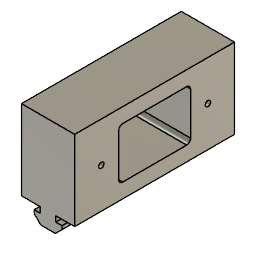
Govde (Autodesk Fusion 360 archive; units mm, degrees)
design "power_soket"
Autodesk Fusion 360 part; units mm, degrees
note: some values were not read from the file. Chosen so that the rebuilt part matches the saved one: which pieces of a blend or face edit are solid.
sketch "Sketch1" plane through (0, 0, 0) normal (0, 1, 0) x (1, 0, 0)
  line L0 (2.8825, -8.6547) -> (4.3945, -10.1667)
  line L1 (3.9, -0.21) -> (3.9, -2.8393)
  line L2 (-8.2, 5.5) -> (-8.2, 3.125)
  line L3 (-2.925, -8.676) -> (-4.4001, -10.1511)
  arc A0 (9.4998, -10.0253) -> (10.0042, -9.4999) centre (9.4925, -9.5135) ccw
  line L4 (0, -4.0611) -> (-0.1019, -4.163)
  line L5 (5.5, 8.2) -> (3.125, 8.2)
  line L6 (-6.5607, -5.5) -> (-8.2, -5.5)
  line L7 (5.2425, -6.658) -> (5.2425, -7.96)
  line L8 (-8.2, -5.5) -> (-8.2, -3.1249)
  line L9 (0, -4.0611) -> (0.1019, -4.163)
  line L10 (-2.7368, -4.163) -> (-5.2537, -6.6799)
  line L11 (-3.125, 8.545) -> (-4.58, 10)
  line L12 (6.5607, 5.5) -> (8.2, 5.5)
  line L13 (-3.125, 8.2) -> (-3.125, 8.545)
  arc A1 (-9.5, 10) -> (-10, 9.5) centre (-9.5, 9.5) ccw
  line L14 (8.2, 3.125) -> (8.545, 3.125)
  line L15 (-3.9, 0.21) -> (-3.9, 2.8393)
  line L16 (-10, 9.5) -> (-10, 4.58)
  line L17 (0.1019, -4.163) -> (2.7475, -4.163)
  line L18 (-3.125, -8.14) -> (-3.125, -8.5931)
  line L19 (-6.5607, 5.5) -> (-8.2, 5.5)
  line L20 (-5.2537, -7.94) -> (-2.925, -7.94)
  line L21 (3.69, 0) -> (3.9, -0.21)
  line L22 (-10.0013, -4.5807) -> (-10.0013, -9.5)
  line L23 (-0.1019, -4.163) -> (-2.7368, -4.163)
  line L24 (-3.69, 0) -> (-3.9, -0.21)
  line L25 (3.9, -2.8393) -> (6.5607, -5.5)
  line L26 (-5.4537, -6.5971) -> (-5.4537, -8.14)
  arc A2 (10, 9.5) -> (9.5, 10) centre (9.5, 9.5) ccw
  line L27 (-3.9, 2.8393) -> (-6.5607, 5.5)
  line L28 (8.545, 3.125) -> (10, 4.58)
  line L29 (10.0042, -4.5823) -> (10.0042, -9.4999)
  line L30 (-5.4537, -8.14) -> (-3.125, -8.14)
  line L31 (-10, -10.0258) -> (-10, -15)
  line L32 (-3.125, -8.5931) -> (-4.5415, -10.0097)
  line L33 (-3.9, -2.8393) -> (-6.5607, -5.5)
  line L34 (3.0825, -8.5719) -> (4.5359, -10.0253)
  line L35 (5.4425, -8.16) -> (3.0825, -8.16)
  line L36 (-2.925, -7.94) -> (-2.925, -8.676)
  line L37 (3.125, 8.2) -> (3.125, 8.545)
  line L38 (8.2, -3.1245) -> (8.5464, -3.1245)
  line L39 (8.2, -5.5) -> (8.2, -3.1245)
  line L40 (0, -3.7782) -> (0.1847, -3.963)
  line L41 (0, -3.7782) -> (-0.1847, -3.963)
  line L42 (0.1847, -3.963) -> (2.8304, -3.963)
  line L43 (-9.5, -10.0097) -> (-4.5415, -10.0097)
  line L44 (4.5359, -10.0253) -> (9.4998, -10.0253)
  line L45 (6.5607, -5.5) -> (8.2, -5.5)
  line L46 (-2.8196, -3.963) -> (-5.4537, -6.5971)
  line L47 (-8.2, -3.1249) -> (-8.5454, -3.1249)
  line L48 (8.5464, -3.1245) -> (10.0042, -4.5823)
  arc A3 (-10.0013, -9.5) -> (-9.5, -10.0097) centre (-9.4969, -9.5053) ccw
  line L49 (10, -15) -> (10, -10.0258)
  line L50 (-5.2537, -6.6799) -> (-5.2537, -7.94)
  line L51 (5.2425, -7.96) -> (2.8825, -7.96)
  line L52 (3.0825, -8.16) -> (3.0825, -8.5719)
  line L53 (5.4425, -6.5751) -> (5.4425, -8.16)
  line L54 (3.9, 0.21) -> (3.9, 2.8393)
  line L55 (-3.9, -0.21) -> (-3.9, -2.8393)
  line L56 (3.9, 2.8393) -> (6.5607, 5.5)
  line L57 (-5.5, 6.5607) -> (-5.5, 8.2)
  line L58 (2.8825, -7.96) -> (2.8825, -8.6547)
  line L59 (-8.5454, -3.1249) -> (-10.0013, -4.5807)
  line L60 (0, 3.69) -> (-0.21, 3.9)
  line L61 (2.8304, -3.963) -> (5.4425, -6.5751)
  line L62 (2.7475, -4.163) -> (5.2425, -6.658)
  line L63 (-8.545, 3.125) -> (-10, 4.58)
  line L64 (-0.1847, -3.963) -> (-2.8196, -3.963)
  line L65 (5.5, 6.5607) -> (5.5, 8.2)
  line L66 (-0.21, 3.9) -> (-2.8393, 3.9)
  line L67 (3.69, 0) -> (3.9, 0.21)
  line L68 (-5.5, 8.2) -> (-3.125, 8.2)
  line L69 (-8.2, 3.125) -> (-8.545, 3.125)
  line L70 (-2.8393, 3.9) -> (-5.5, 6.5607)
  line L71 (2.8393, 3.9) -> (5.5, 6.5607)
  line L72 (10, 9.5) -> (10, 4.58)
  line L73 (8.2, 5.5) -> (8.2, 3.125)
  line L74 (-3.69, 0) -> (-3.9, 0.21)
  line L75 (0.21, 3.9) -> (2.8393, 3.9)
  line L76 (4.58, 10) -> (9.5, 10)
  circle A4 centre (0, 0) radius 2.5
  line L77 (3.125, 8.545) -> (4.58, 10)
  line L78 (-9.5, 10) -> (-4.58, 10)
  line L79 (0, 3.69) -> (0.21, 3.9)
  line L80 (-10, -15) -> (10, -15)
  line L81 (0.1019, -4.163) -> (-0.1019, -4.163)
  line L82 (4.2531, -10.0253) -> (4.5359, -10.0253)
  line L83 (10, -10.0258) -> (4.2536, -10.0258)
  line L84 (-4.2748, -10.0258) -> (-10, -10.0258)
  line L85 (2.8825, -8.6547) -> (2.8825, -10.0258)
  line L86 (2.8825, -10.0258) -> (4.2536, -10.0258)
  line L87 (-2.925, -8.676) -> (-2.925, -10.0353)
  line L88 (-2.925, -10.0353) -> (-4.2748, -10.0258)
  point P0 (0, -10)
  dimension "d1" = 0.2
  dimension "d2" = 5
  constraint parallel L23 L81
  constraint coincident L0 L82.start
  constraint coincident L0 L83.end
  constraint coincident L3 L84.start
  constraint collinear L83 L84
  constraint perpendicular L35 L85
  constraint perpendicular L86 L87
  measures "d2" diameter of A4
extrude "Extrude1" add sketch "Sketch1" along normal blind 60 contours L7 L10 L17 L20 L23 L31 L36 L44 L49 L50 L51 L58 L62 L80 L81 L82 L83 L84 L85 L86 L87 L88
sketch "Sketch2" plane through (10, 0, 0) normal (1, 0, 0) x (0, 1, 0)
  line L0 (0, 15) -> (0, 10.0258)
  line L1 (0, 10.0258) -> (60, 10.0258)
  line L2 (60, 10.0258) -> (60, 15)
  line L3 (60, 15) -> (0, 15)
  line L4 (0, 10.0258) -> (60, 10.0258)
  line L5 (60, 10.0258) -> (60, 40.0258)
  line L6 (60, 40.0258) -> (0, 40.0258)
  line L7 (0, 40.0258) -> (0, 10.0258)
  line L8 (60, 40.0258) -> (0, 10.0258) construction
  line L9 (0, 40.0258) -> (60, 10.0258) construction
  line L10 (43.5, 34.5258) -> (16.5, 34.5258)
  line L11 (16.5, 34.5258) -> (16.5, 15.5258)
  line L12 (16.5, 15.5258) -> (43.5, 15.5258)
  line L13 (43.5, 15.5258) -> (43.5, 34.5258)
  line L14 (43.5, 34.5258) -> (16.5, 15.5258) construction
  line L15 (16.5, 34.5258) -> (43.5, 15.5258) construction
  line L16 (16.5, 25.0258) -> (10, 25.0258)
  line L17 (43.5, 25.0258) -> (50, 25.0258)
  circle A0 centre (10, 25.0258) radius 1
  circle A1 centre (50, 25.0258) radius 1
  point P0 (30, 25.0258)
  dimension "d5" = 30
  dimension "d6" = 60
  dimension "d7" = 27
  dimension "d8" = 19
  dimension "d9" = 6.5
  dimension "d10" = 6.5
  dimension "d11" = 2
  dimension "d12" = 2
  constraint horizontal L4
  constraint vertical L5
  constraint horizontal L6
  constraint vertical L7
  constraint coincident L0.end L1.start
  constraint horizontal L10
  constraint perpendicular L10 L11
  constraint parallel L10 L12
  constraint parallel L11 L13
  constraint coincident L14 P0
  constraint coincident L15 P0
  constraint midpoint L9 P0
  constraint midpoint L11 L16.start
  constraint perpendicular L11 L16
  constraint midpoint L13 L17.start
  constraint perpendicular L13 L17
  constraint coincident L16.end A0.centre
  constraint coincident L17.end A1.centre
  measures "d5" distance of L0.end L6.end
  measures "d6" distance of L5.end L6.end
  measures "d7" distance of L11.end L12.end
  measures "d8" distance of L10.end L11.end
  measures "d9" distance of L16.start L16.end
  measures "d10" distance of L17.start L17.end
  measures "d11" diameter of A0
  measures "d12" diameter of A1
extrude "Extrude2" add sketch "Sketch2" against normal blind 20 contours L3 L5 L6 L7
fillet "Fillet1" radius 1.5 4 edges at (0, 43.5, 15.5258) (0, 16.5, 15.5258) (0, 43.5, 34.5258) (0, 16.5, 34.5258)

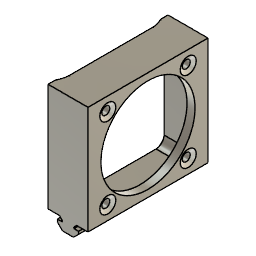
design "fan_duck"
Autodesk Fusion 360 part; units mm, degrees
sketch "Sketch1" plane through (0, 0, 0) normal (0, 1, 0) x (1, 0, 0)
  line L0 (2.925, -8.6278) -> (4.4386, -10.1414)
  line L1 (3.9, -0.21) -> (3.9, -2.8393)
  line L2 (-8.2, 5.5) -> (-8.2, 3.125)
  line L3 (-2.925, -8.6278) -> (-4.4386, -10.1414)
  arc A0 (9.5, -10) -> (10, -9.5) centre (9.5, -9.5) ccw
  line L4 (0, -3.9728) -> (-0.1272, -4.1)
  line L5 (5.5, 8.2) -> (3.125, 8.2)
  line L6 (-6.5607, -5.5) -> (-8.2, -5.5)
  line L7 (5.3, -6.6435) -> (5.3, -8)
  line L8 (-8.2, -5.5) -> (-8.2, -3.125)
  line L9 (0, -3.9728) -> (0.1272, -4.1)
  line L10 (-2.7565, -4.1) -> (-5.3, -6.6435)
  line L11 (-3.125, 8.545) -> (-4.58, 10)
  line L12 (6.5607, 5.5) -> (8.2, 5.5)
  line L13 (-3.125, 8.2) -> (-3.125, 8.545)
  arc A1 (-9.5, 10) -> (-10, 9.5) centre (-9.5, 9.5) ccw
  line L14 (8.2, 3.125) -> (8.545, 3.125)
  line L15 (-3.9, 0.21) -> (-3.9, 2.8393)
  line L16 (-10, 9.5) -> (-10, 4.58)
  line L17 (0.1272, -4.1) -> (2.7565, -4.1)
  line L18 (-3.125, -8.2) -> (-3.125, -8.545)
  line L19 (-6.5607, 5.5) -> (-8.2, 5.5)
  line L20 (-5.3, -8) -> (-2.925, -8)
  line L21 (3.69, 0) -> (3.9, -0.21)
  line L22 (-10, -4.58) -> (-10, -9.5)
  line L23 (-0.1272, -4.1) -> (-2.7565, -4.1)
  line L24 (-3.69, 0) -> (-3.9, -0.21)
  line L25 (3.9, -2.8393) -> (6.5607, -5.5)
  line L26 (-5.5, -6.5607) -> (-5.5, -8.2)
  arc A2 (10, 9.5) -> (9.5, 10) centre (9.5, 9.5) ccw
  line L27 (-3.9, 2.8393) -> (-6.5607, 5.5)
  line L28 (8.545, 3.125) -> (10, 4.58)
  line L29 (10, -4.58) -> (10, -9.5)
  line L30 (-5.5, -8.2) -> (-3.125, -8.2)
  line L31 (-10, -10) -> (-10, -12)
  line L32 (-3.125, -8.545) -> (-4.58, -10)
  line L33 (-3.9, -2.8393) -> (-6.5607, -5.5)
  line L34 (3.125, -8.545) -> (4.58, -10)
  line L35 (5.5, -8.2) -> (3.125, -8.2)
  line L36 (-2.925, -8) -> (-2.925, -8.6278)
  line L37 (3.125, 8.2) -> (3.125, 8.545)
  line L38 (8.2, -3.125) -> (8.545, -3.125)
  line L39 (8.2, -5.5) -> (8.2, -3.125)
  line L40 (0, -3.69) -> (0.21, -3.9)
  line L41 (0, -3.69) -> (-0.21, -3.9)
  line L42 (0.21, -3.9) -> (2.8393, -3.9)
  line L43 (-9.5, -10) -> (-4.58, -10)
  line L44 (4.58, -10) -> (9.5, -10)
  line L45 (6.5607, -5.5) -> (8.2, -5.5)
  line L46 (-2.8393, -3.9) -> (-5.5, -6.5607)
  line L47 (-8.2, -3.125) -> (-8.545, -3.125)
  line L48 (8.545, -3.125) -> (10, -4.58)
  arc A3 (-10, -9.5) -> (-9.5, -10) centre (-9.5, -9.5) ccw
  line L49 (10, -12) -> (10, -10)
  line L50 (-5.3, -6.6435) -> (-5.3, -8)
  line L51 (5.3, -8) -> (2.925, -8)
  line L52 (3.125, -8.2) -> (3.125, -8.545)
  line L53 (5.5, -6.5607) -> (5.5, -8.2)
  line L54 (3.9, 0.21) -> (3.9, 2.8393)
  line L55 (-3.9, -0.21) -> (-3.9, -2.8393)
  line L56 (3.9, 2.8393) -> (6.5607, 5.5)
  line L57 (-5.5, 6.5607) -> (-5.5, 8.2)
  line L58 (2.925, -8) -> (2.925, -8.6278)
  line L59 (-8.545, -3.125) -> (-10, -4.58)
  line L60 (0, 3.69) -> (-0.21, 3.9)
  line L61 (2.8393, -3.9) -> (5.5, -6.5607)
  line L62 (2.7565, -4.1) -> (5.3, -6.6435)
  line L63 (-8.545, 3.125) -> (-10, 4.58)
  line L64 (-0.21, -3.9) -> (-2.8393, -3.9)
  line L65 (5.5, 6.5607) -> (5.5, 8.2)
  line L66 (-0.21, 3.9) -> (-2.8393, 3.9)
  line L67 (3.69, 0) -> (3.9, 0.21)
  line L68 (-5.5, 8.2) -> (-3.125, 8.2)
  line L69 (-8.2, 3.125) -> (-8.545, 3.125)
  line L70 (-2.8393, 3.9) -> (-5.5, 6.5607)
  line L71 (2.8393, 3.9) -> (5.5, 6.5607)
  line L72 (10, 9.5) -> (10, 4.58)
  line L73 (8.2, 5.5) -> (8.2, 3.125)
  line L74 (-3.69, 0) -> (-3.9, 0.21)
  line L75 (0.21, 3.9) -> (2.8393, 3.9)
  line L76 (4.58, 10) -> (9.5, 10)
  circle A4 centre (0, 0) radius 2.5
  line L77 (3.125, 8.545) -> (4.58, 10)
  line L78 (-9.5, 10) -> (-4.58, 10)
  line L79 (0, 3.69) -> (0.21, 3.9)
  line L80 (-10, -12) -> (10, -12)
  line L81 (10, -10) -> (-10, -10)
  line L82 (-4.58, -10) -> (4.58, -10)
  line L83 (0.1272, -4.1) -> (-0.1272, -4.1)
  point P0 (0, -10)
  dimension "d1" = 0.2
  dimension "d2" = 5
  dimension "d3" = 2
  constraint parallel L44 L82
  constraint parallel L23 L83
  measures "d2" diameter of A4
  measures "d3" distance of L49.end L49.start
extrude "Extrude1" add sketch "Sketch1" along normal blind 60 contours L0 L3 L7 L10 L17 L20 L23 L36 L50 L51 L58 L62 L81 L82 L83 | L31 L43 L44 L49 L80 L81 L82
sketch "Sketch2" plane through (10, 0, 0) normal (1, 0, 0) x (0, 1, 0)
  line L0 (0, 12) -> (0, 10)
  line L1 (0, 10) -> (60, 10)
  line L2 (60, 10) -> (60, 12)
  line L3 (60, 12) -> (0, 12)
  line L4 (0, 10) -> (60, 10)
  line L5 (60, 10) -> (60, 64)
  line L6 (60, 64) -> (0, 64)
  line L7 (0, 64) -> (0, 10)
  line L8 (0, 10) -> (60, 64) construction
  line L9 (55, 62) -> (5, 62)
  line L10 (5, 62) -> (5, 12)
  line L11 (5, 12) -> (55, 12)
  line L12 (55, 12) -> (55, 62)
  line L13 (55, 62) -> (5, 12) construction
  line L14 (5, 62) -> (55, 12) construction
  point P0 (30, 37)
  dimension "d6" = 60
  dimension "d7" = 54
  dimension "d8" = 50
  dimension "d9" = 50
  constraint horizontal L4
  constraint vertical L5
  constraint horizontal L6
  constraint vertical L7
  constraint coincident L0.end L1.start
  constraint horizontal L9
  constraint perpendicular L9 L10
  constraint parallel L9 L11
  constraint parallel L10 L12
  constraint coincident L13 P0
  constraint coincident L14 P0
  constraint midpoint L8 P0
  measures "d6" distance of L0.end L1.end
  measures "d7" distance of L0.end L6.end
  measures "d8" distance of L10.end L11.end
  measures "d9" distance of L9.end L10.end
extrude "Extrude2" add sketch "Sketch2" against normal blind 20 contours L3 L5 L6 L7 L9 L10 L12
fillet "Fillet1" radius 4 4 edges at (0, 55, 12) (0, 5, 12) (0, 5, 62) (0, 55, 62)
sketch "Sketch3" plane through (10, 0, 0) normal (1, 0, 0) x (0, 1, 0)
  line L0 (0, 64) -> (0, 10)
  line L1 (0, 10) -> (60, 10)
  line L2 (60, 10) -> (60, 64)
  line L3 (60, 64) -> (0, 64)
  arc A0 (55, 58) -> (51, 62) centre (51, 58) ccw
  line L4 (55, 58) -> (55, 16)
  arc A1 (51, 12) -> (55, 16) centre (51, 16) ccw
  line L5 (51, 12) -> (9, 12)
  arc A2 (5, 16) -> (9, 12) centre (9, 16) ccw
  line L6 (5, 16) -> (5, 58)
  arc A3 (9, 62) -> (5, 58) centre (9, 58) ccw
  line L7 (9, 62) -> (51, 62)
  line L8 (0, 10) -> (60, 64) construction
  line L9 (50.1, 57.1) -> (9.9, 57.1)
  line L10 (9.9, 57.1) -> (9.9, 16.9)
  line L11 (9.9, 16.9) -> (50.1, 16.9)
  line L12 (50.1, 16.9) -> (50.1, 57.1)
  line L13 (50.1, 57.1) -> (9.9, 16.9) construction
  line L14 (9.9, 57.1) -> (50.1, 16.9) construction
  circle A4 centre (50.1, 57.1) radius 2
  circle A5 centre (9.9, 57.1) radius 2
  circle A6 centre (50.1, 16.9) radius 2
  circle A7 centre (9.9, 16.9) radius 2
  circle A8 centre (30, 37) radius 23.5
  point P0 (30, 37)
  dimension "d14" = 40.2
  dimension "d15" = 40.2
  dimension "d16" = 4
  dimension "d17" = 4
  dimension "d18" = 4
  dimension "d19" = 4
  dimension "d20" = 47
  constraint coincident L0.end L1.start
  constraint coincident L2.end L3.start
  constraint horizontal L9
  constraint perpendicular L9 L10
  constraint parallel L9 L11
  constraint parallel L10 L12
  constraint coincident L13 P0
  constraint coincident L14 P0
  constraint midpoint L8 P0
  constraint coincident L9.start L12.end
  constraint coincident L9.end L10.start
  constraint coincident L11.end L12.start
  constraint coincident L10.end L11.start
  constraint coincident P0 A8.centre
  measures "d14" distance of L10.end L11.end
  measures "d15" distance of L9.end L10.end
  measures "d16" diameter of A4
  measures "d17" diameter of A5
  measures "d18" diameter of A6
  measures "d19" diameter of A7
  measures "d20" diameter of A8
extrude "Extrude3" add sketch "Sketch3" against normal blind 4 contours A0 L4 A1 L5 A2 L6 A3 L7 | L9 L10 A5 A8 | L9 L12 A4 A8 | L10 L11 A7 A8 | L11 L12 A6 A8
chamfer "Chamfer1" distance 2 distance2 1 4 edges at (10, 48.2353, 17.6232) (10, 8.0353, 17.6232) (10, 48.2353, 57.8232) (10, 8.0353, 57.8232) measured on face at (10, 2.1667, 37) measured on face at (10, 2.1667, 37) measured on face at (10, 2.1667, 37) measured on face at (10, 2.1667, 37)
chamfer "Chamfer2" distance 4 distance2 3 8 edges at (-10, 55, 37) (-10, 53.8284, 60.8284) (-10, 30, 62) (-10, 6.1716, 60.8284) (-10, 5, 37) (-10, 6.1716, 13.1716) (-10, 30, 12) (-10, 53.8284, 13.1716) measured on face at (-10, 58.3333, 30) measured on face at (0.6667, 51.1903, 61.9955) measured on face at (-10, 58.3333, 30) measured on face at (-4.6667, 5.0181, 58.3802) measured on face at (-10, 58.3333, 30) measured on face at (0.6667, 5.1128, 15.057) measured on face at (-10, 58.3333, 30) measured on face at (0.6667, 51.943, 12.1128)
